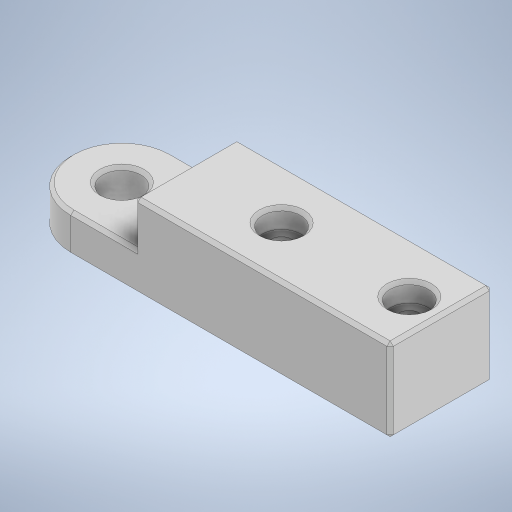
# Autodesk Inventor part: middle_joint
Saved by Autodesk Inventor 2023.1 (Build 271208000, 208)
## iProperties
Created: 2023-11-20
Part Number: middle_joint
Material: Všeobecné
Document SubType Name: Modeling
Designer: zavrel
Density: 1 g/cm^3
Appearance: Výchozí
Author: zavrel
Autodesk Inventor part; units mm, degrees
ref_plane "YZ Plane" through (0, 0, 0) normal (1, 0, 0) x (0, 1, 0)
ref_plane "XZ Plane" through (0, 0, 0) normal (0, 1, 0) x (-1, 0, 0)
ref_plane "XY Plane" through (0, 0, 0) normal (0, 0, 1) x (1, 0, 0)
sketch "Náčrt1" plane through (0, 0, 0) normal (0, 1, 0) x (-1, 0, 0)
  circle A0 centre (0, 0) radius 8
  line L0 (0, -8) -> (-50, -8)
  line L1 (-50, -8) -> (-50, 8)
  line L2 (-50, 8) -> (0, 8)
  circle A1 centre (0, 0) radius 3
  circle A2 centre (0, 0) radius 7.5 construction
  dimension "d0" = 6
  dimension "d1" = 15
  dimension "d2" = 16
  dimension "d3" = 50
  constraints: 6 end point, 3 centre point, 3 coincident, 2 perpendicular, 2 point on circle, 1 horizontal
  measures "d0" diameter of A1
  measures "d1" diameter of A2
  measures "d2" diameter of A0
  measures "d3" distance from line of L1 point (0, 0)
extrude "Vysunutí1" add sketch "Náčrt1" along normal blind 6
sketch "Náčrt2" plane through (0, 6, 0) normal (0, 1, 0) x (1, 0, 0)
  line L0 (0, -8) -> (50, -8) projected
  line L1 (50, -8) -> (50, 8) projected
  line L2 (50, 8) -> (0, 8) projected
  arc A0 (0, 8) -> (0, -8) centre (0, 0) ccw projected
  circle A1 centre (0, 0) radius 3 projected
  circle A2 centre (45, 0) radius 1.6
  circle A3 centre (25, 0) radius 1.6
  dimension "d6" = 5
  dimension "d7" = 25
  dimension "d8" = 3.2
  constraints: 2 centre point, 1 equal radius
  measures "d6" distance from line of L1 A2.centre
  measures "d7" distance from line of L1 A3.centre
  measures "d8" diameter of A3
extrude "Vysunutí2" cut sketch "Náčrt2" against normal through all contours A2 | A3
sketch "Náčrt5" plane through (0, 6, 0) normal (0, 1, 0) x (1, 0, 0)
  circle A0 centre (45, 0) radius 1.6 projected
  circle A1 centre (25, 0) radius 1.6 projected
  line L0 (0, -8) -> (50, -8) projected
  line L1 (50, -8) -> (50, 8) projected
  line L2 (50, 8) -> (0, 8) projected
  arc A2 (0, 8) -> (0, -8) centre (0, 0) ccw projected
  circle A3 centre (0, 0) radius 3 projected
  line L3 (20, 8) -> (20, -8)
  dimension "d19" = 30
  constraints: 2 end point, 2 point on line, 1 vertical
  measures "d19" distance between parallel lines of L1 L3
extrude "Vysunutí5" add sketch "Náčrt5" along normal blind 7 contours L3 L2 L1 L0
sketch "Náčrt7" plane through (0, 13, 0) normal (0, 1, 0) x (1, 0, 0)
  line L0 (50, 8) -> (20, 8) projected
  line L1 (20, 8) -> (20, -8) projected
  line L2 (20, -8) -> (50, -8) projected
  line L3 (50, -8) -> (50, 8) projected
  circle A0 centre (25, 0) radius 1.6 projected
  circle A1 centre (45, 0) radius 1.6 projected
  circle A2 centre (25, 0) radius 1.6 projected
  circle A3 centre (25, 0) radius 3
  circle A4 centre (45, 0) radius 1.6 projected
  circle A5 centre (45, 0) radius 3
  point P0 (0, 0)
  dimension "d22" = 6
  constraints: 2 centre point, 2 coincident, 1 equal radius
  measures "d22" diameter of A3
extrude "Vysunutí6" cut sketch "Náčrt7" against normal blind 3 contours A3 | A5
sketch "Sketch10" plane through (20, 6, -8) normal (-1, 0, 0) x (0, 0, 1)
  line L0 (16, 0) -> (0, 0) projected
  line L1 (16, 0) -> (16, 7) projected
  line L2 (0, 7) -> (16, 7) projected
  line L3 (0, 0) -> (0, 7) projected
  point P0 (8, -6)
extrude "Extrusion8" add sketch "Sketch10" along normal blind 10
chamfer "Chamfer3" distance 0.5 angle 45 21 edges at (5, 6, 8) (-8, 6, 0) (5, 6, -8) (25, 0, 8) (-8, 0, 0) (25, 0, -8) (10, 13, 0) (30, 13, 8) (10, 9.5, 8) (30, 13, -8) (50, 13, 0) (42, 13, 0) (22, 13, 0) (3, 6, 0) (50, 0, 0) (50, 6.5, -8) (50, 6.5, 8) (10, 9.5, -8) (3, 0, 0) (23.4, 0, 0) (43.4, 0, 0)
